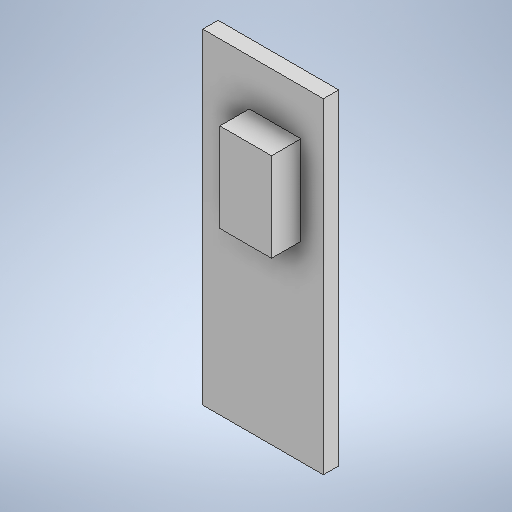
# Autodesk Inventor part: PScaled Modelart2
Saved by Autodesk Inventor 2026.2 (Build 302298010, 298A)
## iProperties
Created: 2026-05-05
Part Number: PScaled Modelart2
Material: Generic
Document SubType Name: Modeling
Designer: piete
Density: 1 g/cm^3
Appearance: Default
Author: piete
Autodesk Inventor part; units mm, degrees
ref_plane "YZ Plane" through (0, 0, 0) normal (1, 0, 0) x (0, 1, 0)
ref_plane "XZ Plane" through (0, 0, 0) normal (0, 1, 0) x (-1, 0, 0)
ref_plane "XY Plane" through (0, 0, 0) normal (0, 0, 1) x (1, 0, 0)
sketch "Sketch1" plane through (0, 0, 0) normal (1, 0, 0) x (0, 1, 0)
  line L0 (10.261, 0.445) -> (-8.629, 0.445)
  line L1 (-8.629, 0.445) -> (-8.629, -0.445)
  line L2 (-8.629, -0.445) -> (10.261, -0.445)
  line L3 (10.261, -0.445) -> (10.261, 0.445)
  point P0 (0, 0)
  dimension "d0" = 18.89
  dimension "d1" = 0.89
  dimension "d2" = 0.445
  dimension "d3" = 8.629
  constraints: 8 end point, 2 parallel, 1 horizontal, 1 perpendicular
  measures "d0" distance of L2.end L1.end
  measures "d1" distance of L0.end L1.end
  measures "d2" distance from line of point (0, 0) L2
  measures "d3" distance from line of L1 point (0, 0)
extrude "Extrusion1" add sketch "Sketch1" along normal blind 7
sketch "Sketch2" plane through (7, 0, 0) normal (1, 0, 0) x (0, 0, -1)
  line L0 (-2.155, 7.601) -> (-0.445, 7.601)
  line L1 (-0.445, 7.601) -> (-0.445, 2.451)
  line L2 (-0.445, 2.451) -> (-2.155, 2.451)
  line L3 (-2.155, 2.451) -> (-2.155, 7.601)
  line L4 (-0.445, 10.261) -> (-0.445, -8.629) projected
  line L5 (-0.445, -8.629) -> (0.445, -8.629) projected
  point P0 (0, 0)
  dimension "d6" = 5.15
  dimension "d7" = 1.71
  dimension "d8" = 0
  dimension "d9" = 11.08
  constraints: 8 end point, 2 parallel, 1 horizontal, 1 perpendicular
  measures "d6" distance of L0.end L1.end
  measures "d7" distance of L1.end L2.end
  measures "d8" distance between parallel lines of L4 L1
  measures "d9" distance between parallel lines of L5 L2
extrude "Extrusion2" add sketch "Sketch2" against normal blind 4.3
extrude "Extrusion3" cut sketch "Sketch2" against normal blind 1.3
equation "\"d2\" = 0.5 * d1"
body "Solid1"
